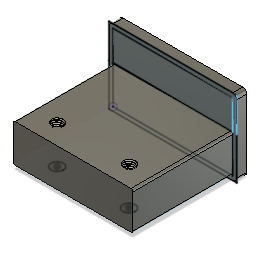
Center Speaker Block (Autodesk Fusion 360 design; units mm, degrees)
Autodesk Fusion 360 part; units mm, degrees
sketch "Sketch1" plane through (0, 0, 0) normal (0, 0, 1) x (1, 0, 0)
  line L0 (0, 0) -> (60, 0)
  line L1 (60, 0) -> (60, 19)
  line L2 (60, 19) -> (0, 19)
  line L3 (0, 19) -> (0, 0)
  line L4 (0, 19) -> (0, 34)
  line L5 (0, 34) -> (60, 34)
  line L6 (60, 34) -> (60, 19)
  line L7 (60, 19) -> (0, 19)
  line L8 (-2, 19) -> (-2, 36)
  line L9 (-2, 36) -> (62, 36)
  line L10 (62, 36) -> (62, 19)
  line L11 (62, -2) -> (62, 19)
  line L12 (-2, -2) -> (62, -2)
  line L13 (-2, 19) -> (-2, -2)
  dimension "d1" = 60
  dimension "d2" = 19
  dimension "d3" = 15
  dimension "d4" = 2
  constraint perpendicular L0 L1
  constraint parallel L0 L2
  constraint parallel L1 L3
  constraint horizontal L0
  constraint coincident L0.start L3.end
  constraint perpendicular L4 L5
  constraint parallel L4 L6
  constraint parallel L5 L7
  constraint perpendicular L2 L4
  measures "d1" distance of L0.start L0.end
  measures "d2" distance of L0.start L2.end
  measures "d3" distance of L2.end L4.end
extrude "Extrude1" add sketch "Sketch1" along normal blind 50 contours L0 L1 L2 L3 L7
extrude "Extrude2" add sketch "Sketch1" against normal blind 5 contours L0 L1 L2 L3 L7 | L2 L4 L5 L6 L7 | L8 L9 L10 L11 L12 L13
sketch "Sketch2" plane through (0, 0, 0) normal (0, -1, 0) x (1, 0, 0)
  line L0 (0, 0) -> (60, 0)
  line L1 (60, 0) -> (60, 50)
  line L2 (60, 50) -> (0, 50)
  line L3 (0, 50) -> (0, 0)
  circle A0 centre (12, 40) radius 3
  circle A1 centre (48, 40) radius 3
  dimension "d11" = 6
  dimension "d12" = 6
  dimension "d13" = 12
  dimension "d14" = 10
  dimension "d15" = 10
  dimension "d16" = 12
  measures "d11" diameter of A0
  measures "d12" diameter of A1
  measures "d13" distance of L3 A0.centre
  measures "d14" distance of L2 A0.centre
  measures "d15" distance of L2 A1.centre
  measures "d16" distance of L1 A1.centre
hole "Hole1" at (12, 0, 40) direction (0, 1, 0) diameter 5.035 end up to surface (19 mm away)
thread "Thread1" "ISO Metric profile 6.0 M6x1 6H" major diameter 6.147 minor diameter 5.035 pitch 1 angle 60 modelled right hand crest width 0.125 on face at (12.2507, 6.3333, 37.495) crest through (12, -0.5625, 37.4825)
hole "Hole2" at (48, 0, 40) direction (0, 1, 0) diameter 5.035 end up to surface (19 mm away)
thread "Thread2" "ISO Metric profile 6.0 M6x1 6H" major diameter 6.147 minor diameter 5.035 pitch 1 angle 60 modelled right hand crest width 0.125 on face at (48.2507, 6.3333, 37.495) crest through (48, -0.5625, 37.4825)
fillet "Fillet1" radius 2 4 edges at (62, 36, -2.5) (-2, 36, -2.5) (62, -2, -2.5) (-2, -2, -2.5)
fillet "Fillet2" radius 1 4 edges at (0, 0, 25) (0, 19, 25) (60, 0, 25) (60, 19, 25)
